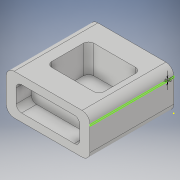
# Autodesk Inventor part: Body EM'
Saved by Autodesk Inventor 2017 (Build 210142000, 142)
## iProperties
Created: 2020-02-13
Part Number: Body EM'
Material: Generic
Document SubType Name: Modeling
Designer: 10042265
Density: 1 g/cm^3
Appearance: Default
Author: 10042265
Autodesk Inventor part; units mm, degrees
ref_plane "YZ Plane" through (0, 0, 0) normal (1, 0, 0) x (0, 1, 0)
ref_plane "XZ Plane" through (0, 0, 0) normal (0, 1, 0) x (-1, 0, 0)
ref_plane "XY Plane" through (0, 0, 0) normal (0, 0, 1) x (1, 0, 0)
sketch "Sketch1" plane through (0, 0, 0) normal (0, 0, 1) x (1, 0, 0)
  line L0 (7.62, 0) -> (72.898, 0)
  line L1 (0, 7.62) -> (0, 31.242)
  line L2 (7.62, 38.862) -> (72.898, 38.862)
  line L3 (80.518, 31.242) -> (80.518, 7.62)
  arc A0 (7.62, 38.862) -> (0, 31.242) centre (7.62, 31.242) ccw
  arc A1 (80.518, 31.242) -> (72.898, 38.862) centre (72.898, 31.242) ccw
  arc A2 (72.898, 0) -> (80.518, 7.62) centre (72.898, 7.62) ccw
  arc A3 (0, 7.62) -> (7.62, 0) centre (7.62, 7.62) ccw
  point P0 (0, 0)
  point P1 (80.518, 0)
  point P2 (0, 38.862)
  dimension "d2" = 80.518
  dimension "d3" = 38.862
  dimension "d4" = 7.62
  dimension "d5" = 7.62
  dimension "d6" = 7.62
  dimension "d7" = 7.62
  constraints: 8 end point, 8 point on circle, 8 tangent, 6 point on line, 4 centre point, 2 perpendicular, 1 horizontal, 1 vertical
  measures "d2" distance of point (0, 0) point (80.518, 0)
  measures "d3" distance of point (0, 0) point (0, 38.862)
  measures "d4" radius of A0
  measures "d5" radius of A1
  measures "d6" radius of A2
  measures "d7" radius of A3
extrude "Extrusion1" add sketch "Sketch1" along normal blind 80.518
sketch "Sketch2" plane through (0, 0, 80.518) normal (0, 0, 1) x (1, 0, 0)
  line L0 (14.732, 7.62) -> (65.532, 7.62)
  line L1 (70.612, 12.7) -> (70.612, 26.162)
  line L2 (65.532, 31.242) -> (14.732, 31.242)
  line L3 (9.652, 26.162) -> (9.652, 12.7)
  arc A0 (14.732, 31.242) -> (9.652, 26.162) centre (14.732, 26.162) ccw
  arc A1 (70.612, 26.162) -> (65.532, 31.242) centre (65.532, 26.162) ccw
  arc A2 (65.532, 7.62) -> (70.612, 12.7) centre (65.532, 12.7) ccw
  arc A3 (9.652, 12.7) -> (14.732, 7.62) centre (14.732, 12.7) ccw
  point P0 (0, 0)
  point P1 (9.652, 7.62)
  point P2 (70.612, 7.62)
  point P3 (70.612, 31.242)
  dimension "d12" = 60.96
  dimension "d13" = 23.622
  dimension "d16" = 5.08
  constraints: 8 end point, 8 point on circle, 8 tangent, 6 point on line, 4 centre point, 3 equal radius, 2 perpendicular, 1 horizontal, 1 vertical
  measures "d12" distance of point (9.652, 7.62) point (70.612, 7.62)
  measures "d13" distance of point (70.612, 7.62) point (70.612, 31.242)
  measures "d16" radius of A0
extrude "Extrusion2" cut sketch "Sketch2" against normal blind 14.478
sketch "Sketch3" plane through (7.62, 38.862, 0) normal (0, 1, 0) x (1, 0, 0)
  line L0 (60.198, -54.2068) -> (60.198, -23.9808)
  line L1 (55.118, -18.9008) -> (14.986, -18.9008)
  line L2 (9.906, -23.9808) -> (9.906, -54.2068)
  line L3 (14.986, -59.2868) -> (55.118, -59.2868)
  line L4 (72.898, 0) -> (72.898, -80.518) projected
  arc A0 (14.986, -18.9008) -> (9.906, -23.9808) centre (14.986, -23.9808) ccw
  arc A1 (60.198, -23.9808) -> (55.118, -18.9008) centre (55.118, -23.9808) ccw
  arc A2 (55.118, -59.2868) -> (60.198, -54.2068) centre (55.118, -54.2068) ccw
  arc A3 (9.906, -54.2068) -> (14.986, -59.2868) centre (14.986, -54.2068) ccw
  point P0 (-7.62, 0)
  point P1 (60.198, -59.2868)
  point P2 (60.198, -18.9008)
  point P3 (9.906, -18.9008)
  point P4 (9.906, -59.2868)
  dimension "d19" = 40.386
  dimension "d20" = 50.292
  dimension "d21" = 12.7
  dimension "d33" = 5.08
  constraints: 8 end point, 8 point on circle, 8 point on line, 8 tangent, 4 centre point, 3 equal radius, 2 perpendicular, 1 horizontal
  measures "d19" distance of point (60.198, -59.287) point (60.198, -18.901)
  measures "d20" distance of point (60.198, -18.901) point (9.906, -18.901)
  measures "d21" distance between parallel lines of L4 L0
  measures "d33" radius of A0
extrude "Extrusion3" cut sketch "Sketch3" against normal blind 27.178
sketch "Sketch4" plane through (0, 0, 0) normal (0, 0, -1) x (-1, 0, 0)
  line L0 (-8.6279, 26.924) -> (-8.6279, 11.684)
  line L1 (-72.1279, 11.684) -> (-72.1279, 26.924)
  line L2 (-67.0479, 32.004) -> (-13.7079, 32.004)
  line L3 (-13.7079, 6.604) -> (-67.0479, 6.604)
  arc A0 (-67.0479, 32.004) -> (-72.1279, 26.924) centre (-67.0479, 26.924) ccw
  arc A1 (-8.6279, 26.924) -> (-13.7079, 32.004) centre (-13.7079, 26.924) ccw
  arc A2 (-13.7079, 6.604) -> (-8.6279, 11.684) centre (-13.7079, 11.684) ccw
  arc A3 (-72.1279, 11.684) -> (-67.0479, 6.604) centre (-67.0479, 11.684) ccw
  point P0 (0, 0)
  point P1 (-8.6279, 32.004)
  point P2 (-8.6279, 6.604)
  point P3 (-72.1279, 6.604)
  point P4 (-72.1279, 32.004)
  dimension "d26" = 25.4
  dimension "d27" = 63.5
  dimension "d29" = 25.4
  dimension "d30" = 5.08
  constraints: 8 end point, 8 point on circle, 8 point on line, 8 tangent, 4 centre point, 3 equal radius, 1 horizontal, 1 perpendicular
  measures "d26" distance of point (-8.628, 32.004) point (-8.628, 6.604)
  measures "d27" distance of point (-8.628, 6.604) point (-72.128, 6.604)
  measures "d29" distance of point (-72.128, 6.604) point (-72.128, 32.004)
  measures "d30" radius of A0
extrude "Extrusion4" cut sketch "Sketch4" against normal blind 14.478
sketch "Sketch5" plane through (80.518, 7.62, 0) normal (1, 0, 0) x (0, 0, -1)
  line L0 (-80.518, 23.622) -> (0, 23.622)
  line L1 (0, 23.622) -> (-80.518, 23.622) projected
  line L2 (0, 23.622) -> (0, 22.098)
  line L3 (0, 22.098) -> (-80.518, 22.098)
  line L4 (-80.518, 23.622) -> (-66.04, 23.622) projected
  line L5 (-80.518, 22.098) -> (-80.518, 23.622)
  line L6 (-80.518, 23.622) -> (-80.518, 22.098)
  point P0 (0, -7.62)
  dimension "d34" = 1.524
  constraints: 10 end point, 2 perpendicular, 1 horizontal
  measures "d34" distance of L0.end L2.end
body "Solid1"
